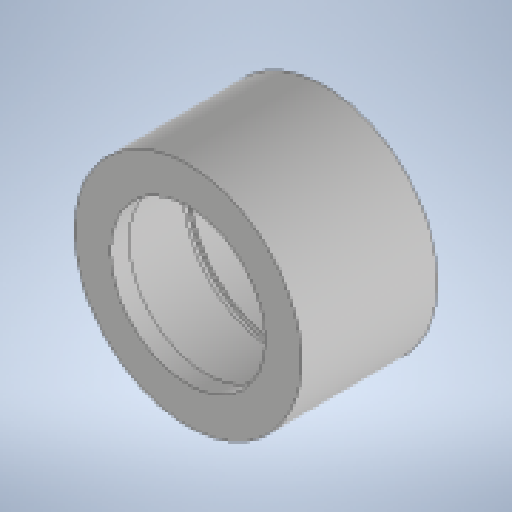
# Autodesk Inventor part: Седло для сальника
Saved by Autodesk Inventor 2025 (Build 290162010, 162A)
## iProperties
Created: 2024-07-07
Part Number: Седло для сальника
Material: Generic
Document SubType Name: Modeling
Designer: pokla
Density: 1 g/cm^3
Appearance: Default
Stock Number: Седло для сальника
Author: pokla
Autodesk Inventor part; units mm, degrees
ref_plane "YZ Plane" through (0, 0, 0) normal (1, 0, 0) x (0, 1, 0)
ref_plane "XZ Plane" through (0, 0, 0) normal (0, 1, 0) x (-1, 0, 0)
ref_plane "XY Plane" through (0, 0, 0) normal (0, 0, 1) x (1, 0, 0)
sketch "Sketch5" plane through (0, 0, 0) normal (0, 0, 1) x (1, 0, 0)
  line L0 (20, 14) -> (25, 14)
  line L1 (25, 14) -> (25, -16)
  line L2 (25, -16) -> (17, -16)
  line L3 (17, -16) -> (17, -12)
  line L4 (17, -12) -> (20, -12)
  line L5 (20, -12) -> (20, 3)
  line L6 (20, 4.6) -> (21, 4.6)
  line L7 (21, 4.6) -> (21, 3)
  line L8 (21, 3) -> (20, 3)
  line L9 (20, 3) -> (20, 4.6)
  line L10 (20, 13.2) -> (21, 13.2)
  line L11 (21, 13.2) -> (21, 11.6)
  line L12 (21, 11.6) -> (20, 11.6)
  line L13 (20, 11.6) -> (20, 13.2)
  line L14 (20, 13.2) -> (20, 14)
  line L15 (20, 11.6) -> (20, 13.2) construction
  line L16 (20, 4.6) -> (20, 11.6)
  line L17 (20, 3) -> (20, 4.6) construction
  line L18 (0, 0) -> (0, 17.2013)
  point P0 (20, 0)
  point P1 (20, 3.8)
  point P2 (20, 12.4)
  dimension "d12" = 30
  dimension "d13" = 4
  dimension "d14" = 3
  dimension "d15" = 25
  dimension "d16" = 5
  dimension "d17" = 1.6
  dimension "d19" = 15
  dimension "d20" = 1
  dimension "d21" = 1
  dimension "d22" = 1.6
  dimension "d23" = 7
  dimension "d24" = 14
  constraints: 38 end point, 11 perpendicular, 4 parallel, 3 horizontal, 2 midpoint, 2 vertical alignment, 1 horizontal alignment, 1 vertical
  measures "d12" distance of L0.end L1.end
  measures "d13" distance of L2.end L3.end
  measures "d14" distance of L3.end L4.end
  measures "d15" distance from line of L1 L18.start
  measures "d16" distance of L0.start L0.end
  measures "d17" distance of L6.end L7.end
  measures "d19" distance of L4.end L5.end
  measures "d20" distance of L6.start L6.end
  measures "d21" distance of L10.start L10.end
  measures "d22" distance of L10.end L11.end
  measures "d23" distance between parallel lines of L6 L12
  measures "d24" distance from line of L18.start L0
revolve "Revolution1" add sketch "Sketch5" angle 360 about axis through (0, 0, 0) along (0, 1, 0)
equation "\"d21\" = d20"
equation "\"d22\" = d17"
body "Solid2"
